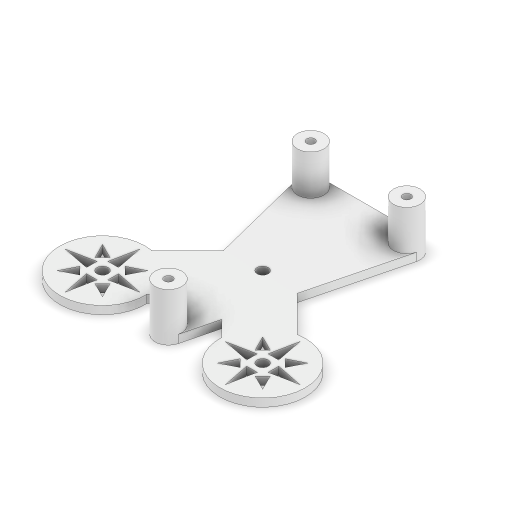
# Autodesk Inventor part: BASE_LIDAR
Saved by Autodesk Inventor 2024.2 (Build 282272000, 272)
## iProperties
Created: 2024-07-17
Part Number: BASE_LIDAR
Material: ABS Plastic
Document SubType Name: Modeling
Designer: jrcer
Density: 1.06 g/cm^3
Appearance: Smooth - White
Author: jrcer
Autodesk Inventor part; units mm, degrees
ref_plane "YZ Plane" through (0, 0, 0) normal (1, 0, 0) x (0, 1, 0)
ref_plane "XZ Plane" through (0, 0, 0) normal (0, 1, 0) x (-1, 0, 0)
ref_plane "XY Plane" through (0, 0, 0) normal (0, 0, 1) x (1, 0, 0)
sketch "Sketch1" plane through (0, 0, 0) normal (0, 1, 0) x (-1, 0, 0)
  circle A0 centre (0, 35.3) radius 1.55
  circle A1 centre (18, -36) radius 1.55
  circle A2 centre (-18, -36) radius 1.55
  circle A3 centre (0, 35.3) radius 5
  circle A4 centre (18, -36) radius 5
  circle A5 centre (-18, -36) radius 5
  point P0 (0, 0)
  dimension "d0" = 35.3
  dimension "d1" = 36
  dimension "d2" = 3.1
  dimension "d3" = 10
  dimension "d4" = 36
  dimension "d5" = 18
  constraints: 6 centre point, 4 equal radius, 3 coincident, 1 horizontal alignment, 1 vertical alignment
  measures "d0" distance of A0.centre point (0, 0)
  measures "d1" vertical distance of A2.centre point (0, 0)
  measures "d2" diameter of A0
  measures "d3" diameter of A3
  measures "d4" distance of A2.centre A1.centre
  measures "d5" horizontal distance of point (0, 0) A2.centre
extrude "Extrusion1" add sketch "Sketch1" along normal blind 15
sketch "Sketch2" plane through (0, 0, 35.3) normal (0, -1, 0) x (1, 0, 0)
  circle A0 centre (0, 0) radius 5 projected
  circle A1 centre (0, 0) radius 1.55 projected
  circle A2 centre (-18, -71.3) radius 1.55 projected
  circle A3 centre (-18, -71.3) radius 5 projected
  circle A4 centre (18, -71.3) radius 1.55 projected
  circle A5 centre (18, -71.3) radius 5 projected
  line L0 (-22.8479, -70.0761) -> (-4.8479, 1.2239)
  line L1 (22.8479, -70.0761) -> (4.8479, 1.2239)
  line L2 (-18, -76.3) -> (18, -76.3)
  circle A6 centre (0, -35.3) radius 2.1
  dimension "d8" = 4.2
  constraints: 6 end point, 6 point on circle, 5 tangent, 1 centre point, 1 coincident, 1 horizontal
  measures "d8" diameter of A6
extrude "Extrusion2" add sketch "Sketch2" along normal blind 3
sketch "Sketch3" plane through (0, 0, 35.3) normal (0, 1, 0) x (1, 0, 0)
  circle A0 centre (-30, 5.3) radius 16
  circle A1 centre (0, 35.3) radius 29.9 construction
  line L0 (0, 35.3) -> (-30, 5.3) construction
  line L1 (0, 35.3) -> (-30, 35.3) construction
  circle A2 centre (-30, 5.3) radius 2.1 construction
  line L2 (-28, 9.3) -> (-32, 9.3)
  line L3 (-32, 9.3) -> (-30, 19.3)
  line L4 (-30, 19.3) -> (-28, 9.3)
  line L5 (-27.9, 5.3) -> (-32.1, 5.3) construction
  line L6 (-30, 3.2) -> (-30, 7.4) construction
  line L7 (-30, 5.3) -> (-30, 35.3) construction
  line L8 (-26, 3.3) -> (-26, 7.3)
  line L9 (-26, 7.3) -> (-16, 5.3)
  line L10 (-16, 5.3) -> (-26, 3.3)
  line L11 (-24.3431, 8.1284) -> (-27.1716, 10.9569)
  line L12 (-27.1716, 10.9569) -> (-21.5147, 13.7853)
  line L13 (-24.3431, 8.1284) -> (-21.5147, 13.7853)
  circle A3 centre (-30, 5.3) radius 2.1
  line L14 (-24.3431, 2.4716) -> (-27.1716, -0.3569)
  line L15 (-27.1716, -0.3569) -> (-21.5147, -3.1853)
  line L16 (-24.3431, 2.4716) -> (-21.5147, -3.1853)
  line L17 (-35.6569, 8.1284) -> (-32.8284, 10.9569)
  line L18 (-32.8284, 10.9569) -> (-38.4853, 13.7853)
  line L19 (-35.6569, 8.1284) -> (-38.4853, 13.7853)
  line L20 (-35.6569, 2.4716) -> (-38.4853, -3.1853)
  line L21 (-32.8284, -0.3569) -> (-38.4853, -3.1853)
  line L22 (-35.6569, 2.4716) -> (-32.8284, -0.3569)
  line L23 (-34, 3.3) -> (-34, 7.3)
  line L24 (-34, 7.3) -> (-44, 5.3)
  line L25 (-44, 5.3) -> (-34, 3.3)
  line L26 (-28, 1.3) -> (-32, 1.3)
  line L27 (-32, 1.3) -> (-30, -8.7)
  line L28 (-30, -8.7) -> (-28, 1.3)
  circle A4 centre (0, 0) radius 5 projected
  line L29 (-4.8479, -1.2239) -> (-22.8479, 70.0761) projected
  line L30 (-13.8479, 34.4261) -> (-27.2178, 21.0562)
  line L31 (-8.1467, 11.8431) -> (-14.0143, 5.9755)
  circle A5 centre (0, 35.3) radius 2.1 construction
  point P0 (-25.7574, 9.5426)
  dimension "d41" = 59.8
  dimension "d49" = 30
  dimension "d50" = 45
  dimension "d51" = 32
  dimension "d52" = 4.2
  dimension "d53" = 4
  dimension "d54" = 10
  dimension "d55" = 4
  dimension "d56" = 4
  dimension "d57" = 4
  dimension "d58" = 6
  dimension "d59" = 6
  dimension "d70" = 20
  dimension "d71" = 45
  constraints: 62 end point, 15 symmetric about line, 6 midpoint, 6 point on circle, 4 centre point, 4 equal length, 3 coincident, 3 horizontal, 3 point on line, 3 vertical, 2 vertical alignment, 1 concentric, 1 horizontal alignment, 1 parallel, 1 perpendicular, 1 other
  measures "d41" diameter of A1
  measures "d49" distance of L0.start L1.end
  measures "d50" angle of L1 L0
  measures "d51" diameter of A0
  measures "d52" diameter of A2
  measures "d53" distance of L2.start L2.end
  measures "d54" distance from line of L3.end L2
  measures "d55" distance from line of L2 L7.start
  measures "d56" distance from line of L0.end L8
  measures "d57" distance of L11.start L11.end
  measures "d58" distance from line of L12.end L11
  measures "d59" distance from line of L0.end L11
  measures "d70" distance between parallel lines of L30 L31
  measures "d71" angle of L1 L30
extrude "Extrusion3" add sketch "Sketch3" against normal blind 3 contours A0 | A0 L30 L29 L31
mirror "Mirror1" about plane through (0, 0, 0) normal (1, 0, 0) of "Extrusion3"
equation "\"d5\" = 0.5 * d4"
body "Solid1"
